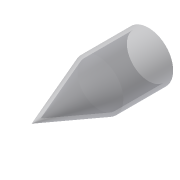
# Autodesk Inventor part: FalconTube15mL
Saved by Autodesk Inventor 2014 (Build 180170000, 170)
## iProperties
Created: 2016-07-07
Part Number: FalconTube15mL
Material: Generic
Document SubType Name: Modeling
Designer: Camilo
Density: 1 g/cm^3
Appearance: Polycarbonate - Clear
Author: Camilo
Autodesk Inventor part; units mm, degrees
ref_plane "YZ Plane" through (0, 0, 0) normal (1, 0, 0) x (0, 1, 0)
ref_plane "XZ Plane" through (0, 0, 0) normal (0, 1, 0) x (-1, 0, 0)
ref_plane "XY Plane" through (0, 0, 0) normal (0, 0, 1) x (1, 0, 0)
sketch "Sketch1" plane through (0, 0, 0) normal (0, 1, 0) x (-1, 0, 0)
  circle A0 centre (0, 0) radius 7.925
  dimension "d5" = 15.85
  constraints: 1 centre point, 1 coincident
  measures "d5" diameter of A0
extrude "Extrusion1" add sketch "Sketch1" along normal blind 16
sketch "Sketch2" plane through (0, 0, 0) normal (1, 0, 0) x (0, 1, 0)
  line L0 (16, -7.925) -> (16, 7.925) projected
  line L1 (0, 7.925) -> (0, -7.925) projected
  line L2 (0, 7.925) -> (0, -7.925) projected
  line L3 (0, 7.925) -> (-21.5, 0)
  line L4 (-21.5, 0) -> (0, 0)
  line L5 (0, 7.925) -> (0, 0)
  dimension "d2" = 21.5
  constraints: 6 end point
  measures "d2" distance of L3.end L4.end
revolve "Revolution1" add sketch "Sketch2" angle 360 about axis through (0, -21.5, 0) along (0, 1, 0)
shell "Shell1" thickness 1 removed faces 1 at (2.2031, 16, 0.1081)
body "Solid1"
